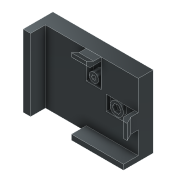
# Autodesk Inventor part: Catcher
Saved by Autodesk Inventor 2021 (Build 250183000, 183)
## iProperties
Created: 2025-07-03
Part Number: Catcher
Material: Generic
Document SubType Name: Modeling
Designer: Owner
Density: 1 g/cm^3
Appearance: Iron Gray
Author: Owner
Autodesk Inventor part; units mm, degrees
ref_plane "YZ Plane" through (0, 0, 0) normal (1, 0, 0) x (0, 1, 0)
ref_plane "XZ Plane" through (0, 0, 0) normal (0, 1, 0) x (-1, 0, 0)
ref_plane "XY Plane" through (0, 0, 0) normal (0, 0, 1) x (1, 0, 0)
sketch "Sketch1" plane through (0, 0, 0) normal (0, 0, 1) x (1, 0, 0)
  line L0 (-5.75, -4) -> (5.75, -4)
  line L1 (5.75, -4) -> (5.75, 4)
  line L2 (5.75, 4) -> (-5.75, 4)
  line L3 (-5.75, 4) -> (-5.75, -4)
  line L4 (-5.75, -4) -> (5.75, 4) construction
  line L5 (5.75, -4) -> (-5.75, 4) construction
  line L6 (-6.75, -5.5) -> (6.75, -5.5)
  line L7 (6.75, -5.5) -> (6.75, 5.5)
  line L8 (6.75, 5.5) -> (-6.75, 5.5)
  line L9 (-6.75, 5.5) -> (-6.75, -5.5)
  line L10 (-6.75, -5.5) -> (6.75, 5.5) construction
  line L11 (6.75, -5.5) -> (-6.75, 5.5) construction
  point P0 (0, 0)
  dimension "d0" = 11.5
  dimension "d1" = 8
  dimension "d2" = 13.5
  dimension "d3" = 11
  constraints: 24 end point, 4 midpoint, 4 parallel, 2 horizontal, 2 perpendicular
  measures "d0" distance of L2.end L1.end
  measures "d1" distance of L1.end L0.end
  measures "d2" distance of L8.end L7.end
  measures "d3" distance of L7.end L6.end
extrude "Extrusion1" add sketch "Sketch1" along normal blind 2
sketch "Sketch2" plane through (0, 0, 0) normal (0, 0, -1) x (-1, 0, 0)
  line L0 (-5.75, -4.5) -> (5.75, -4.5)
  line L1 (5.75, -4.5) -> (5.75, 3.5)
  line L2 (5.75, 3.5) -> (-5.75, 3.5)
  line L3 (-5.75, 3.5) -> (-5.75, -4.5)
  line L4 (-5.75, -4.5) -> (5.75, 3.5) construction
  line L5 (5.75, -4.5) -> (-5.75, 3.5) construction
  line L6 (-6.75, -6) -> (6.75, -6)
  line L7 (6.75, -6) -> (6.75, 5)
  line L8 (6.75, 5) -> (-6.75, 5)
  line L9 (-6.75, 5) -> (-6.75, -6)
  line L10 (-6.75, -6) -> (6.75, 5) construction
  line L11 (6.75, -6) -> (-6.75, 5) construction
  point P0 (0, 0)
  point P1 (0, -0.5)
  dimension "d6" = 11.5
  dimension "d7" = 8
  dimension "d8" = 13.5
  dimension "d9" = 11
  constraints: 24 end point, 4 midpoint, 4 parallel, 2 horizontal, 2 perpendicular
  measures "d6" distance of L2.end L1.end
  measures "d7" distance of L1.end L0.end
  measures "d8" distance of L8.end L7.end
  measures "d9" distance of L7.end L6.end
extrude "Extrusion2" add sketch "Sketch2" along normal blind 2 contours L3 L2 L1 L0 | L9 L8 L7 L6
sketch "Sketch3" plane through (0, 0, 2) normal (0, 0, 1) x (1, 0, 0)
  line L0 (6.75, -5.5) -> (6.75, 5.5) projected
  line L1 (5.75, -4) -> (6.75, -4)
  line L2 (6.75, -4) -> (6.75, -1.5)
  line L3 (6.75, -1.5) -> (5.75, -1.5)
  line L4 (5.75, -1.5) -> (5.75, -4)
  line L5 (5.75, 4) -> (5.75, -4) projected
  line L6 (5.75, 4) -> (6.75, 4)
  line L7 (6.75, 4) -> (6.75, 1.5)
  line L8 (6.75, 1.5) -> (5.75, 1.5)
  line L9 (5.75, 1.5) -> (5.75, 4)
  point P0 (0, 0)
  dimension "d12" = 2.5
  dimension "d13" = 2.5
  constraints: 16 end point, 4 parallel, 2 horizontal, 2 perpendicular, 2 point on line
  measures "d12" distance of L2.end L1.end
  measures "d13" distance of L6.end L7.end
extrude "Extrusion3" cut sketch "Sketch3" against normal blind 2 contours L1 L4 L3 L0 | L8 L5 L6 L0
sketch "Sketch4" plane through (0, 0, 2) normal (0, 0, 1) x (1, 0, 0)
  line L0 (6.75, 5.5) -> (-6.75, 5.5) projected
  line L1 (-5.75, 4) -> (-0.25, 4)
  line L2 (-0.25, 4) -> (-0.25, 5.5)
  line L3 (-0.25, 5.5) -> (-5.75, 5.5)
  line L4 (-5.75, 5.5) -> (-5.75, 4)
  line L5 (-6.75, -5.5) -> (6.75, -5.5) projected
  line L6 (-5.75, -4) -> (-0.25, -4)
  line L7 (-0.25, -4) -> (-0.25, -5.5)
  line L8 (-0.25, -5.5) -> (-5.75, -5.5)
  line L9 (-5.75, -5.5) -> (-5.75, -4)
  line L10 (-5.75, 4) -> (6.75, 4) projected
  line L11 (1.75, 4) -> (6.7628, 4)
  line L12 (6.7628, 4) -> (6.7628, 5.5)
  line L13 (6.7628, 5.5) -> (1.75, 5.5)
  line L14 (1.75, 5.5) -> (1.75, 4)
  point P0 (0, 0)
  point P1 (1.75, 5.5)
  point P2 (6.75, 4)
  point P3 (-5.75, 5.5)
  dimension "d16" = 5.5
  dimension "d17" = 5.5
  dimension "d18" = 2
  constraints: 24 end point, 6 parallel, 4 point on line, 3 horizontal, 3 perpendicular
  measures "d16" distance of L3.end L2.end
  measures "d17" distance of L7.end L8.end
  measures "d18" distance between parallel lines of L14 L2
extrude "Extrusion4" cut sketch "Sketch4" against normal blind 2 contours L13 L12 L11 L10 L14 L0 | L2 L1 L4 L0 | L9 L6 L7 L5
sketch "Sketch5" plane through (0, 0, 0) normal (0, 0, 1) x (1, 0, 0)
  line L0 (-6.75, -6) -> (-6.75, 5) projected
  line L1 (6.75, -5.5) -> (6.75, -6) projected
  line L2 (-6.75, -6) -> (6.75, -6)
  line L3 (6.75, -6) -> (6.75, -5.5)
  line L4 (6.75, -5.5) -> (-6.75, -5.5)
  line L5 (-6.75, -5.5) -> (-6.75, -6)
  point P0 (0, 0)
  point P1 (-6.75, -5.5)
  constraints: 8 end point, 2 parallel, 1 horizontal, 1 perpendicular
extrude "Extrusion5" cut sketch "Sketch5" against normal blind 2
sketch "Sketch6" plane through (0, 0, 0) normal (0, 0, -1) x (-1, 0, 0)
  line L0 (-1.75, 4) -> (-1.75, 5) projected
  line L1 (-1.75, 5.5) -> (0.25, 5.5) projected
  line L2 (-1.75, 5) -> (0.25, 5)
  line L3 (0.25, 5) -> (0.25, 5.5)
  line L4 (0.25, 5.5) -> (-1.75, 5.5)
  line L5 (-1.75, 5.5) -> (-1.75, 5)
  point P0 (0, 0)
  constraints: 8 end point, 2 parallel, 1 horizontal, 1 perpendicular
extrude "Extrusion6" cut sketch "Sketch6" against normal blind 2
sketch "Sketch7" plane through (0, 0, 0) normal (0, 0, -1) x (-1, 0, 0)
  line L0 (0.25, 5) -> (5.75, 5) projected
  line L1 (6.75, 5.5) -> (6.75, -5.5) projected
  line L2 (5.75, 5) -> (6.75, 5)
  line L3 (6.75, 5) -> (6.75, 5.5)
  line L4 (6.75, 5.5) -> (5.75, 5.5)
  line L5 (5.75, 5.5) -> (5.75, 5)
  point P0 (0, 0)
  constraints: 8 end point, 2 parallel, 1 horizontal, 1 perpendicular
extrude "Extrusion7" cut sketch "Sketch7" against normal blind 2
sketch "Sketch8" plane through (0, 0, 0) normal (0, 0, 1) x (1, 0, 0)
  line L0 (5.75, 1.5) -> (5.75, -1.5) projected
  line L1 (5.75, -1.5) -> (5.75, 1.5)
  line L2 (-0.25, 4) -> (1.75, 4) projected
  line L3 (1.75, 4) -> (-0.25, 4)
  line L4 (-0.25, 4) -> (-0.25, 1.2)
  line L5 (-0.25, 1.2) -> (1.75, 1.2)
  line L6 (1.75, 1.2) -> (1.75, 4)
  line L7 (5.75, -1) -> (2.45, -1)
  line L8 (2.45, -1) -> (2.45, 1)
  line L9 (2.45, 1) -> (5.75, 1)
  line L10 (5.75, 1) -> (5.75, -1)
  line L11 (6.75, 1.5) -> (5.75, 1.5) projected
  line L12 (5.75, -1.5) -> (6.75, -1.5) projected
  point P0 (0, 0)
  dimension "d28" = 2.8
  dimension "d57" = 3.3
  dimension "d58" = 2
  dimension "d59" = 0.5
  dimension "d60" = 0.5
  constraints: 18 end point, 4 parallel, 2 horizontal, 2 perpendicular, 1 point on line
  measures "d28" distance of L4.end L3.end
  measures "d57" distance of L8.end L9.end
  measures "d58" distance of L7.end L8.end
  measures "d59" distance between parallel lines of L11 L9
  measures "d60" distance between parallel lines of L12 L7
extrude "Extrusion8" cut sketch "Sketch8" against normal blind 1 contours L2 L6 L5 L4
sketch "Sketch9" plane through (0, 0, -1) normal (0, 0, 1) x (1, 0, 0)
  circle A0 centre (0.75, 2.0964) radius 0.6413
  point P0 (0, 0)
  constraints: 1 centre point
extrude "Extrusion9" add sketch "Sketch9" along normal blind 1
sketch "Sketch10" plane through (0, 0, -1) normal (0, 0, 1) x (1, 0, 0)
  circle A0 centre (4.0861, 0) radius 0.75
  point P0 (0, 0)
  dimension "d33" = 1.5
  constraints: 1 centre point
  measures "d33" diameter of A0
extrude "Extrusion10" add sketch "Sketch10" along normal blind 1
sketch "Sketch11" plane through (4.0861, 0, 0) normal (0, 0, 1) x (1, 0, 0)
  line L0 (0.1861, -0.3022) -> (-0.1686, -0.3123)
  line L1 (-0.1686, -0.3123) -> (-0.3547, -0.0101)
  line L2 (-0.3547, -0.0101) -> (-0.1861, 0.3022)
  line L3 (-0.1861, 0.3022) -> (0.1686, 0.3123)
  line L4 (0.1686, 0.3123) -> (0.3547, 0.0101)
  line L5 (0.3547, 0.0101) -> (0.1861, -0.3022)
  point P0 (-4.0861, 0)
  point P1 (0, 0)
  constraints: 12 end point, 13 other
extrude "Extrusion11" cut sketch "Sketch11" against normal blind 0.5
sketch "Sketch12" plane through (0.75, 2.0964, 0) normal (0, 0, 1) x (1, 0, 0)
  circle A0 centre (0, 0) radius 0.6413 projected
  line L0 (0.1462, -0.2589) -> (-0.1511, -0.2561)
  line L1 (-0.1511, -0.2561) -> (-0.2973, 0.0028)
  line L2 (-0.2973, 0.0028) -> (-0.1462, 0.2589)
  line L3 (-0.1462, 0.2589) -> (0.1511, 0.2561)
  line L4 (0.1511, 0.2561) -> (0.2973, -0.0028)
  line L5 (0.2973, -0.0028) -> (0.1462, -0.2589)
  point P0 (-0.75, -2.0964)
  constraints: 12 end point, 1 coincident, 13 other
extrude "Extrusion12" cut sketch "Sketch12" against normal blind 0.5 contours L0 L1 L2 L3 L4 L5
sketch "Sketch13" plane through (6.75, -5.5, 2) normal (1, 0, 0) x (0, 0, -1)
  line L0 (0, 4) -> (2, 4) projected
  line L1 (0.5, 4) -> (-0.5, 4)
  line L2 (-0.5, 4) -> (-0.5, 7)
  line L3 (-0.5, 7) -> (0.5, 7)
  line L4 (0.5, 7) -> (0.5, 4)
  line L5 (2, 10.5) -> (2, 7) projected
  point P0 (2, 5.5)
  dimension "d40" = 1
  dimension "d41" = 1.5
  constraints: 8 end point, 2 parallel, 1 horizontal, 1 perpendicular, 1 point on line
  measures "d40" distance of L2.end L3.end
  measures "d41" distance between parallel lines of L5 L4
extrude "Extrusion13" add sketch "Sketch13" along normal blind 0.5
sketch "Sketch14" plane through (5.75, 1.5, 0) normal (0, 1, 0) x (1, 0, 0)
  line L0 (1, 0) -> (1, -1.5) projected
  line L1 (1, 0) -> (1, -1)
  line L2 (1, -1) -> (1.5, -2)
  line L3 (1.5, -1.5) -> (1.5, -2.5) projected
  line L4 (0, -2) -> (1, -2) projected
  line L5 (1, -2) -> (1.5, -2)
  line L6 (0, 0) -> (1, 0) projected
  line L7 (0.5, 0) -> (0.5, -1.5)
  line L8 (0.5, -1.5) -> (1, -2)
  point P0 (-5.75, 0)
  dimension "d44" = 1
  constraints: 10 end point, 2 midpoint, 1 perpendicular, 1 point on line, 1 vertical
  measures "d44" distance of L0.start L1.end
extrude "Extrusion14" add sketch "Sketch14" along normal blind 5
sketch "Sketch15" plane through (5.75, -1.5, 0) normal (0, -1, 0) x (1, 0, 0)
  line L0 (0, 2) -> (1, 2) projected
  line L1 (0, 0) -> (0, 2) projected
  line L2 (0, 0) -> (1, 0) projected
  line L3 (1, 1.5) -> (1, 0) projected
  line L4 (1, 1.5) -> (1.5, 1.5) projected
  line L5 (1.5, 2.5) -> (1.5, 1.5) projected
  line L6 (1, 2.5) -> (1.5, 2.5) projected
  line L7 (1, 2.5) -> (1, 2) projected
  point P0 (-5.75, 0)
extrude "Extrusion15" cut sketch "Sketch15" against normal blind 3
sketch "Sketch16" plane through (5.75, 1.5, 0) normal (0, -1, 0) x (1, 0, 0)
  line L0 (1, 1) -> (1.5, 2) projected
  line L1 (1.5, 2) -> (1, 2) projected
  line L2 (1, 2) -> (0.5, 1.5) projected
  line L3 (0.5, 1.5) -> (0.5, 0) projected
  line L4 (1, 0) -> (0.5, 0) projected
  line L5 (1, 1) -> (1, 0) projected
  point P0 (-5.75, 0)
extrude "Extrusion16" add sketch "Sketch16" along normal blind 3
sketch "Sketch17" plane through (5.75, 6.5, 0) normal (0, 1, 0) x (1, 0, 0)
  line L0 (1, -2) -> (1.5, -2) projected
  line L1 (1.5, -2) -> (1, -1) projected
  line L2 (1, -1) -> (1, 0) projected
  line L3 (1, 0) -> (0.5, 0) projected
  line L4 (0.5, 0) -> (0.5, -1.5) projected
  line L5 (0.5, -1.5) -> (1, -2) projected
  point P0 (-5.75, 0)
extrude "Extrusion17" cut sketch "Sketch17" against normal blind 5
sketch "Sketch18" plane through (5.75, 1.5, 0) normal (0, 1, 0) x (1, 0, 0)
  line L0 (1, -1) -> (1.5, -2) projected
  line L1 (1, 0) -> (1, -1) projected
  line L2 (0.5, 0) -> (1, 0) projected
  line L3 (0.5, -1.5) -> (0.5, 0) projected
  line L4 (1, -2) -> (0.5, -1.5) projected
  line L5 (1.5, -2) -> (1, -2) projected
  point P0 (-5.75, 0)
extrude "Extrusion18" cut sketch "Sketch18" against normal blind 0.5
sketch "Sketch19" plane through (5.75, -1.5, 0) normal (0, -1, 0) x (1, 0, 0)
  line L0 (1, 1) -> (1.5, 2) projected
  line L1 (1.5, 2) -> (1, 2) projected
  line L2 (1, 2) -> (0.5, 1.5) projected
  line L3 (0.5, 1.5) -> (0.5, 0) projected
  line L4 (1, 0) -> (0.5, 0) projected
  line L5 (1, 0) -> (1, 1) projected
  point P0 (-5.75, 0)
extrude "Extrusion19" cut sketch "Sketch19" against normal blind 0.5
sketch "Sketch20" plane through (0, 0, 0) normal (0, 0, 1) x (1, 0, 0)
  line L0 (6.25, -1) -> (6.25, 1) projected
  line L1 (6.25, -1) -> (2.45, -1)
  line L2 (2.45, -1) -> (2.45, 1)
  line L3 (2.45, 1) -> (6.25, 1)
  line L4 (6.25, 1) -> (6.25, -1)
  point P0 (0, 0)
  dimension "d61" = 3.8
  dimension "d62" = 2
  constraints: 8 end point, 2 parallel, 1 horizontal, 1 perpendicular
  measures "d61" distance of L2.end L3.end
  measures "d62" distance of L1.end L2.end
extrude "Extrusion20" cut sketch "Sketch20" against normal blind 0.5
sketch "Sketch21" plane through (4.0861, 0, -0.5) normal (0, 0, 1) x (1, 0, 0)
  circle A0 centre (-0.2528, 0) radius 0.8942
  point P0 (-4.0861, 0)
  constraints: 1 centre point
extrude "Extrusion21" add sketch "Sketch21" along normal blind 0.5
sketch "Sketch22" plane through (3.8333, 0, 0) normal (0, 0, 1) x (1, 0, 0)
  line L0 (0.5864, 0) -> (0.2932, -0.5078)
  line L1 (0.2932, -0.5078) -> (-0.2932, -0.5078)
  line L2 (-0.2932, -0.5078) -> (-0.5864, 0)
  line L3 (-0.5864, 0) -> (-0.2932, 0.5078)
  line L4 (-0.2932, 0.5078) -> (0.2932, 0.5078)
  line L5 (0.2932, 0.5078) -> (0.5864, 0)
  point P0 (-3.8333, 0)
  point P1 (0, 0)
  constraints: 12 end point, 13 other
extrude "Extrusion22" cut sketch "Sketch22" against normal blind 0.5
sketch "Sketch23" plane through (-6.75, 5, -2) normal (0, 1, 0) x (1, 0, 0)
  line L0 (8.5, -4) -> (6.5, -4) projected
  line L1 (6.5, -4) -> (6.5, -2) projected
  line L2 (8.5, -4) -> (6.5, -4)
  line L3 (6.5, -4) -> (6.5, -3)
  line L4 (6.5, -3) -> (8.5, -3)
  line L5 (8.5, -3) -> (8.5, -4)
  point P0 (6.75, -2)
  dimension "d69" = 1
  constraints: 8 end point, 2 parallel, 1 horizontal, 1 midpoint, 1 perpendicular
  measures "d69" distance of L2.end L3.end
extrude "Extrusion23" add sketch "Sketch23" along normal blind 0.5
sketch "Sketch24" plane through (-0.25, 4, 0) normal (-1, 0, 0) x (0, 0, 1)
  line L0 (2, 1.0059) -> (2.0029, 1.5059)
  line L1 (2.0029, 1.5059) -> (1, 1.0118)
  line L2 (1, 1.0118) -> (0.0057, 1.0176)
  line L3 (0.0057, 1.0176) -> (0, 0.5177)
  line L4 (0, 0.5177) -> (1.4999, 0.5005)
  line L5 (1.4999, 0.5005) -> (2, 1.0059)
  line L6 (2, 1.5) -> (2, 0) projected
  line L7 (2, 1.0059) -> (2, 0)
  line L8 (0, 0) -> (-1, 0) projected
  line L9 (2, 0) -> (0, 0)
  line L10 (0, 0) -> (0, 0.5177)
  point P0 (0, -4)
  point P1 (-5.75, 0)
  constraints: 18 end point, 2 perpendicular, 1 vertical
extrude "Extrusion24" add sketch "Sketch24" along normal blind 4 contours L5 L4 L3 L2 L1 L0
sketch "Sketch25" plane through (1.75, 4, 0) normal (1, 0, 0) x (0, 0, -1)
  line L0 (0, 1) -> (-1, 1) projected
  line L1 (-1, 1) -> (-1, 1.5) projected
  line L2 (-2, 1.5) -> (-1, 1.5) projected
  line L3 (-2, 0) -> (-2, 1.5) projected
  line L4 (0, 0) -> (-2, 0) projected
  line L5 (0, 0) -> (0, 1) projected
  point P0 (0, -4)
extrude "Extrusion25" cut sketch "Sketch25" against normal blind 2
sketch "Sketch26" plane through (-0.25, 4, 0) normal (1, 0, 0) x (0, 0, -1)
  line L0 (-2.0029, 1.5059) -> (-1, 1.0118) projected
  line L1 (-2, 1.0059) -> (-2.0029, 1.5059) projected
  line L2 (-2, 1.0059) -> (-1.4999, 0.5005) projected
  line L3 (-1.4999, 0.5005) -> (0, 0.5177) projected
  line L4 (0, 0.5177) -> (-0.0057, 1.0176) projected
  line L5 (-0.0057, 1.0176) -> (-1, 1.0118) projected
  point P0 (0, -4)
extrude "Extrusion26" add sketch "Sketch26" along normal blind 2
sketch "Sketch27" plane through (-4.25, 4, 0) normal (-1, 0, 0) x (0, 0, 1)
  line L0 (1.4999, 0.5005) -> (0, 0.5177) projected
  line L1 (0, 0.5177) -> (0.0057, 1.0176) projected
  line L2 (0.0057, 1.0176) -> (1, 1.0118) projected
  line L3 (1, 1.0118) -> (2.0029, 1.5059) projected
  line L4 (2.0029, 1.5059) -> (2, 1.0059) projected
  line L5 (2, 1.0059) -> (1.4999, 0.5005) projected
  point P0 (0, -4)
extrude "Extrusion27" cut sketch "Sketch27" against normal blind 4
sketch "Sketch28" plane through (0, 0, 0) normal (0, 0, 1) x (1, 0, 0)
  line L0 (-0.25, 1.2) -> (-0.25, 4) projected
  line L1 (1.75, 4.5177) -> (1.75, 5.0176) projected
  line L2 (-0.25, 4) -> (1.75, 4)
  line L3 (1.75, 4) -> (1.75, 4.5177)
  line L4 (1.75, 4.5177) -> (-0.25, 4.5177)
  line L5 (-0.25, 4.5177) -> (-0.25, 4)
  point P0 (0, 0)
  constraints: 8 end point, 2 parallel, 1 horizontal, 1 perpendicular
extrude "Extrusion28" cut sketch "Sketch28" against normal blind 1
sketch "Sketch29" plane through (-6.75, -5.5, 2) normal (0, -1, 0) x (1, 0, 0)
  line L0 (1, -2) -> (1, 0) projected
  line L1 (0, 0) -> (1, 0) projected
  line L2 (0, -4) -> (0, 0) projected
  line L3 (13.5, -4) -> (0, -4) projected
  line L4 (13.5, 0) -> (13.5, -4) projected
  line L5 (6.5, 0) -> (13.5, 0) projected
  line L6 (6.5, 0) -> (6.5, -2) projected
  line L7 (1, -2) -> (6.5, -2) projected
  point P0 (6.75, -2)
extrude "Extrusion29" cut sketch "Sketch29" against normal blind 0.5
sketch "Sketch30" plane through (-6.75, -5, 2) normal (0, -1, 0) x (1, 0, 0)
  line L0 (1, -2) -> (6.5, -2) projected
  line L1 (1, 0) -> (1, -2) projected
  line L2 (0, 0) -> (1, 0) projected
  line L3 (0, -4) -> (0, 0) projected
  line L4 (13.5, -4) -> (0, -4) projected
  line L5 (13.5, 0) -> (13.5, -4) projected
  line L6 (6.5, 0) -> (13.5, 0) projected
  line L7 (6.5, -2) -> (6.5, 0) projected
  point P0 (6.75, -2)
extrude "Extrusion30" cut sketch "Sketch30" against normal blind 0.3
body "Solid1"
